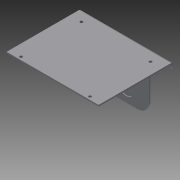
# Autodesk Inventor part: backplate
Saved by Autodesk Inventor 2013 (Build 170138000, 138)
## iProperties
Created: 2012-12-03
Part Number: backplate
Material: Generic
Document SubType Name: Sheet Metal
Designer: Istvan
Density: 1 g/cm^3
Sheet Metal Rule: Default
Author: Istvan
Autodesk Inventor part; units mm, degrees
ref_plane "YZ Plane" through (0, 0, 0) normal (1, 0, 0) x (0, 1, 0)
ref_plane "XZ Plane" through (0, 0, 0) normal (0, 1, 0) x (-1, 0, 0)
ref_plane "XY Plane" through (0, 0, 0) normal (0, 0, 1) x (1, 0, 0)
sketch "Sketch1" plane through (0, 0, 0) normal (0, 1, 0) x (-1, 0, 0)
  line L0 (0, 0) -> (203.2, 0)
  line L1 (203.2, 0) -> (203.2, 165.1)
  line L2 (203.2, 165.1) -> (0, 165.1)
  line L3 (0, 165.1) -> (0, 0)
  dimension "d0" = 203.2
  dimension "d1" = 165.1
  measures "d0" distance of L2.end L1.end
  measures "d1" distance of L1.end L0.end
extrude "Plate2" add sketch "Sketch1" along normal blind 3.048
sketch "Sketch4" plane through (0, 3.048, 3.048) normal (0, 0, -1) x (-1, 0, 0)
  line L0 (203.2, 0) -> (0, 0)
  line L1 (0, 0) -> (0, -127)
  line L2 (0, -127) -> (203.2, -127)
  line L3 (203.2, -127) -> (203.2, 0)
  constraints: 6 end point, 1 horizontal, 1 perpendicular, 1 vertical
edge flange "Flange1" height 127 angle 90 thickness 3.048 bend radius 3.048 thickness toward (0, 0, -1) relief straight relief width 3.048 relief depth 1.524 edges at (-101.6, 0, 0) wall of the first edge with corners at (-203.2, 3.048, 3.048) (0, 3.048, 3.048) (0, -123.952, 3.048) (-203.2, -123.952, 3.048)
bend "Bend1"
corner "Corner1"
sketch "Sketch5" plane through (0, 3.048, 0) normal (0, 1, 0) x (1, 0, 0)
  line L0 (0, -6.096) -> (-203.2, -6.096) projected
  line L1 (-203.2, -165.1) -> (-203.2, -6.096) projected
  line L2 (0, -6.096) -> (0, -165.1) projected
  point P0 (0, 0)
  point P1 (-177.8, -25.146)
  point P2 (-25.4, -25.146)
  point P3 (-25.4, -158.496)
  point P4 (-177.8, -158.496)
  dimension "d27" = 25.4
  dimension "d28" = 25.4
  dimension "d29" = 19.05
  dimension "d30" = 133.35
  constraints: 2 horizontal alignment, 2 vertical alignment
  measures "d27" distance from line of L1 point (-177.8, -25.146)
  measures "d28" distance from line of L2 point (-25.4, -25.146)
  measures "d29" distance from line of L0 point (-177.8, -25.146)
  measures "d30" distance of point (-177.8, -158.496) point (-177.8, -25.146)
hole "Hole2" at (-177.8, 3.048, 25.146) at (-25.4, 3.048, 25.146) at (-25.4, 3.048, 158.496) at (-177.8, 3.048, 158.496) direction (0, -1, 0) diameter 6.35 end through all
sketch "Sketch6" plane through (0, -123.952, 0) normal (0, 0, -1) x (-1, 0, 0)
  line L0 (203.2, 120.904) -> (0, 120.904) projected
  line L1 (0, 0) -> (0, 120.904) projected
  line L2 (203.2, 0) -> (0, 0) projected
  line L3 (203.2, 120.904) -> (203.2, 0) projected
  line L4 (50.8, 120.904) -> (152.4, 120.904)
  line L5 (152.4, 70.104) -> (152.4, 25.4)
  line L6 (127, 0) -> (76.2, 0)
  line L7 (50.8, 25.4) -> (50.8, 70.104)
  arc A0 (50.8, 25.4) -> (76.2, 0) centre (76.2, 25.4) ccw
  arc A1 (127, 0) -> (152.4, 25.4) centre (127, 25.4) ccw
  line L8 (12.7, 108.204) -> (12.7, 108.204)
  line L9 (0, 0) -> (0, 108.204)
  line L10 (0, 0) -> (76.2, 0)
  line L11 (203.2, 0) -> (127, 0)
  line L12 (190.5, 108.204) -> (190.5, 108.204)
  line L13 (203.2, 108.204) -> (203.2, 0)
  arc A2 (50.8, 70.104) -> (12.7, 108.204) centre (12.7, 70.104) ccw
  arc A3 (190.5, 108.204) -> (152.4, 70.104) centre (190.5, 70.104) ccw
  line L14 (0, 120.904) -> (0, 120.904)
  line L15 (203.2, 120.904) -> (203.2, 120.904)
  arc A4 (190.5, 108.204) -> (203.2, 120.904) centre (190.5, 120.904) ccw
  arc A5 (0, 120.904) -> (12.7, 108.204) centre (12.7, 120.904) ccw
  point P0 (0, 123.952)
  point P1 (152.4, 0)
  point P2 (50.8, 0)
  dimension "d38" = 101.6
  dimension "d40" = 50.8
  dimension "d41" = 50.8
  dimension "d42" = 25.4
  dimension "d43" = 12.7
  dimension "d44" = 38.1
  dimension "d47" = 12.7
  constraints: 24 end point, 14 point on line, 14 tangent, 12 point on circle, 6 centre point, 6 collinear, 4 perpendicular, 3 equal radius, 2 parallel, 1 horizontal
  measures "d38" distance of point (152.4, 0) point (50.8, 0)
  measures "d40" distance between parallel lines of L1 L7
  measures "d41" distance between parallel lines of L3 L5
  measures "d42" radius of A0
  measures "d43" distance between parallel lines of L0 L8
  measures "d44" radius of A2
  measures "d47" radius of A4
extrude "Extrusion2" cut sketch "Sketch6" against normal through all contours L3 L2 A1 L5 A3 A4 | A5 A2 L7 A0 L2 L1
sketch "Sketch8" plane through (-203.2, -3.048, 3.048) normal (0, 0, 1) x (1, 0, 0)
  line L0 (76.2, -120.904) -> (127, -120.904) projected
  line L1 (152.4, -95.504) -> (152.4, -50.8) projected
  line L2 (50.8, -50.8) -> (50.8, -95.504) projected
  circle A0 centre (101.6, -89.154) radius 19.05
  point P0 (203.2, 3.048)
  dimension "d53" = 38.1
  dimension "d54" = 50.8
  dimension "d55" = 50.8
  dimension "d56" = 31.75
  constraints: 1 centre point, 1 coincident
  measures "d53" diameter of A0
  measures "d54" distance from line of L2 point (101.6, -89.154)
  measures "d55" distance from line of L1 point (101.6, -89.154)
  measures "d56" distance from line of L0 point (101.6, -89.154)
extrude "Extrusion3" cut sketch "Sketch8" against normal blind 1.524
sketch "Sketch9" plane through (-101.6, -92.202, 1.524) normal (0, 0, 1) x (1, 0, 0)
  circle A0 centre (0, 0) radius 19.05 projected
  circle A1 centre (0, 0) radius 3.81
  point P0 (101.6, 92.202)
  dimension "d59" = 7.62
  constraints: 3 coincident, 1 centre point
  measures "d59" diameter of A1
extrude "Extrusion4" cut sketch "Sketch9" against normal through all contours A1
equation "\"d40\" = d41"
equation "\"d17\" = BendReliefWidth"
equation "\"d18\" = BendReliefDepth"
equation "\"d19\" = MinimumRemnant"
equation "\"d20\" = BendRadius"
equation "\"d23\" = BendRadius"
equation "\"d24\" = CornerReliefSize"
equation "\"d25\" = GapSize"
equation "\"d26\" = JacobiRadiusSize"
equation "\"d54\" = d55"
equation "\"BendRadius\" = Thickness"
equation "\"BendReliefWidth\" = Thickness"
equation "\"BendReliefDepth\" = 0.5 * Thickness"
equation "\"CornerReliefSize\" = 4 * Thickness"
equation "\"MinimumRemnant\" = 2 * Thickness"
equation "\"TransitionRadius\" = BendRadius"
equation "\"JacobiRadiusSize\" = Thickness"
equation "\"GapSize\" = Thickness"
equation "\"d15\" = BendRadius"
equation "\"d16\" = BendRadius"
equation "\"Thickness\" = 3.048"
body "Solid2"
